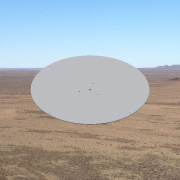
# Autodesk Inventor part: 2f1bd
Saved by Autodesk Inventor 2014 SP1 (Build 180222100, 222)
## iProperties
Company: HERA Project
Created: 2013-05-22
Part Number: 2f1bd
Material: Aluminum 6061
Document SubType Name: Modeling
Designer: Rich Bradley
Density: 2.71 g/cm^3
Description: Feed bottom disk
Mass: 2472.03 g
Surface Area: 5814.47 cm^2
Volume: 912.187 cm^3
Appearance: Aluminum - Flat
Translation Standard: STEP AP214IS
FileName: C:/Users/Dave/Desktop/PAPER/paperElement.step
PostProcessor: Build: 138, Release: 2013 RTM - Date: Thu 03/01/2012
Sent Units: millimeter
Uncertainty: 2.54e-05
Author: David DeBoer
Title: Feed bottom disk
Autodesk Inventor part; units mm, degrees
ref_plane "YZ Plane" through (0, 0, 0) normal (1, 0, 0) x (0, 1, 0)
ref_plane "XZ Plane" through (0, 0, 0) normal (0, 1, 0) x (-1, 0, 0)
ref_plane "XY Plane" through (0, 0, 0) normal (0, 0, 1) x (1, 0, 0)
sketch "Sketch1" plane through (0, 0, 0) normal (0, 1, 0) x (-1, 0, 0)
  circle A0 centre (0, 0) radius 304.8
  dimension "d0" = 609.6
  constraints: 1 centre point, 1 coincident
  measures "d0" diameter of A0
extrude "Extrusion1" add sketch "Sketch1" along normal blind 3.175
sketch "Sketch2" plane through (0, 3.175, 0) normal (0, 1, 0) x (1, 0, 0)
  circle A0 centre (0, 0) radius 304.8 projected
  circle A1 centre (0, 0) radius 6.35
  dimension "d3" = 12.7
  constraints: 1 centre point, 1 coincident
  measures "d3" diameter of A1
extrude "Extrusion2" cut sketch "Sketch2" against normal blind 3.175 contours A1
sketch "Sketch3" plane through (0, 3.175, 0) normal (0, 1, 0) x (1, 0, 0)
  circle A0 centre (0, 0) radius 6.35 projected
  circle A1 centre (0, 292.1) radius 4.6302
  dimension "d6" = 292.1
  constraints: 1 centre point
  measures "d6" distance of A1.centre A0.centre
hole "Hole1" at (0, 3.175, -292.1) direction (0, -1, 0) diameter 4.4958 end through all countersink diameter 8.4328 countersink angle 82
pattern_circular "Circular Pattern1" count 4 over 360 about axis through (0, 3.175, 0) along (0, -1, 0) of "Hole1"
sketch "Sketch7" plane through (0, 3.175, 0) normal (0, 1, 0) x (1, 0, 0)
  circle A0 centre (0, 0) radius 304.8 projected
  line L0 (0, 0) -> (57.15, 0) construction
  circle A1 centre (57.15, 0) radius 2.1123
  dimension "d60" = 57.15
  constraints: 2 end point, 1 centre point, 1 coincident, 1 horizontal
  measures "d60" distance of L0.start L0.end
hole "Hole5" at (57.15, 3.175, 0) direction (0, -1, 0) diameter 6.756 depth 8 tip angle 118 clearance for "Flat Head Machine Screw (82)" size "1/4" standard "Ansi Unified Screw Threads"
pattern_circular "Circular Pattern6" count 3 over 360 about axis through (0, 3.175, 0) along (0, -1, 0) of "Hole5"
body "Solid2"
